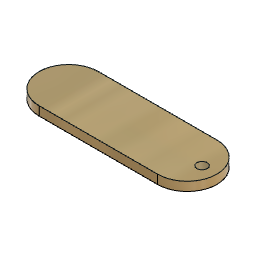
keytag_blank (Autodesk Fusion 360 design; units mm, degrees)
Autodesk Fusion 360 part; units mm, degrees
sketch "Sketch1" plane through (0, 0, 0) normal (0, 0, 1) x (1, 0, 0)
  line L0 (0, 0) -> (40, 0) construction
  line L1 (0, 10) -> (40, 10)
  line L2 (0, -10) -> (40, -10)
  arc A0 (0, 10) -> (0, -10) centre (0, 0) ccw
  arc A1 (40, -10) -> (40, 10) centre (40, 0) ccw
  circle A2 centre (45, 0) radius 1.75
  line L3 (50, 9.724) -> (50, -11.0876) construction
  dimension "d1" = 20
  dimension "d2" = 20
  dimension "d3" = 40
  dimension "d4" = 3.5
  dimension "d5" = 5
  constraint coincident L0.start A0.centre
  constraint coincident L0.end A1.centre
  constraint horizontal L0
  constraint horizontal L1
  constraint tangent L1 A0
  constraint horizontal L2
  constraint tangent L2 A0
  constraint vertical L3
  constraint tangent A1 L3
  measures "d1" diameter of A0
  measures "d2" diameter of A1
  measures "d3" distance of L0.start L0.end
  measures "d4" diameter of A2
  measures "d5" distance of A2.centre L3
extrude "Extrude1" add sketch "Sketch1" along normal blind 3
sketch "DXF_outline" plane through (0, 0, 3) normal (0, 0, 1) x (-1, 0, 0)
  circle A0 centre (-45, 0) radius 1.75
  arc A1 (0, -10) -> (0, 10) centre (0, 0) ccw
  line L0 (0, 10) -> (-40, 10)
  arc A2 (-40, 10) -> (-40, -10) centre (-40, 0) ccw
  line L1 (-40, -10) -> (0, -10)
equation "d1 = width"
equation "d2 = d1"
equation "d3 = length"
equation "d4 = keyhole"
equation "d5 = d4 + 1.5 mm"
equation "width = 20 mm" comment "Width"
equation "length = 40 mm" comment "Overall length"
equation "keyhole = 3.5 mm" comment "Key hole diameter"
